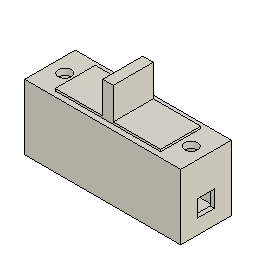
Fuse holder RT14 v0 (Autodesk Fusion 360 design; units mm, degrees)
Autodesk Fusion 360 part; units mm, degrees
sketch "Sketch1" plane through (0, 0, 0) normal (0, 0, 1) x (1, 0, 0)
  line L0 (35, -10) -> (-35, -10)
  line L1 (-35, -10) -> (-35, 10)
  line L2 (-35, 10) -> (35, 10)
  line L3 (35, 10) -> (35, -10)
  line L4 (35, -10) -> (-35, 10) construction
  line L5 (-35, -10) -> (35, 10) construction
  dimension "d1" = 70
  dimension "d2" = 20
  constraint horizontal L0
  constraint perpendicular L0 L1
  constraint parallel L0 L2
  constraint parallel L1 L3
  constraint coincident L4 origin
  constraint coincident L5 origin
  measures "d1" distance of L1.end L2.end
extrude "Extrude1" add sketch "Sketch1" along normal blind 29
sketch "Sketch2" plane through (0, 0, 0) normal (0, 0, -1) x (1, 0, 0)
  line L0 (-35, -10) -> (35, -10)
  line L1 (35, -10) -> (35, 10)
  line L2 (35, 10) -> (-35, 10)
  line L3 (-35, 10) -> (-35, -10)
  circle A0 centre (0, 0) radius 2.25
  dimension "d5" = 4.5
  constraint coincident A0.centre origin
  measures "d5" diameter of A0
shell "Shell1" thickness 2 outward yes removed faces 1 at (11.6667, -3.3333, 29)
extrude "Extrude2" cut sketch "Sketch2" along normal blind 6.615 contours A0
sketch "Sketch3" plane through (-37, 0, 0) normal (-1, 0, 0) x (0, -1, 0)
  line L0 (-12, -2) -> (12, -2)
  line L1 (12, -2) -> (12, 29)
  line L2 (12, 29) -> (-12, 29)
  line L3 (-12, 29) -> (-12, -2)
  line L4 (-4, 13) -> (4, 13)
  line L5 (4, 13) -> (4, 5)
  line L6 (4, 5) -> (-4, 5)
  line L7 (-4, 5) -> (-4, 13)
  line L8 (0, 13) -> (0, 29) construction
  dimension "d9" = 8
  dimension "d10" = 16
  constraint horizontal L4
  constraint vertical L5
  constraint horizontal L6
  constraint vertical L7
  constraint midpoint L4 L8.start
  constraint perpendicular L4 L8
  constraint equal L4 L5
  constraint midpoint L2 L8.end
  measures "d9" distance of L4.start L4.end
  measures "d10" distance of L8.start L8.end
extrude "Extrude3" cut sketch "Sketch3" against normal blind 131.311 contours L4 L5 L6 L7
sketch "Sketch4" plane through (0, 0, 29) normal (0, 0, 1) x (-1, 0, 0)
  line L0 (-35, -10) -> (-35, 10)
  line L1 (-35, 10) -> (35, 10)
  line L2 (35, 10) -> (35, -10)
  line L3 (35, -10) -> (-35, -10)
  line L4 (-37, -12) -> (37, -12)
  line L5 (37, -12) -> (37, 12)
  line L6 (37, 12) -> (-37, 12)
  line L7 (-37, 12) -> (-37, -12)
  line L8 (35, -10) -> (-35, -10)
  line L9 (-35, -10) -> (-35, 10)
  line L10 (-35, 10) -> (35, 10)
  line L11 (35, 10) -> (35, -10)
  circle A0 centre (30, 0) radius 3
  circle A1 centre (-30, 0) radius 3
  line L12 (-22, 7) -> (22, 7)
  line L13 (22, 7) -> (22, -7)
  line L14 (22, -7) -> (-22, -7)
  line L15 (-22, -7) -> (-22, 7)
  line L16 (-22, 7) -> (22, -7) construction
  line L17 (22, 7) -> (-22, -7) construction
  line L18 (30, 0) -> (-30, 0) construction
  dimension "d13" = 6
  dimension "d14" = 60
  dimension "d15" = 44
  dimension "d16" = 14
  constraint horizontal L8
  constraint vertical L9
  constraint horizontal L10
  constraint vertical L11
  constraint coincident L0.end L1.start
  constraint coincident L2.end L3.start
  constraint horizontal L12
  constraint perpendicular L12 L13
  constraint parallel L12 L14
  constraint parallel L13 L15
  constraint coincident L16 origin
  constraint coincident L17 origin
  constraint equal A0 A1
  constraint coincident A0.centre L18.start
  constraint coincident A1.centre L18.end
  constraint perpendicular L15 L18
  constraint midpoint origin L18
  measures "d13" diameter of A0
  measures "d14" distance of A0.centre A1.centre
  measures "d15" distance of L13.end L14.end
  measures "d16" distance of L12.start L14.end
extrude "Extrude4" add sketch "Sketch4" against normal blind 3 contours L0 L1 L2 L3 L8 L9 L10 L11
sketch "Sketch5" plane through (0, 0, 29) normal (0, 0, 1) x (-1, 0, 0)
  circle A0 centre (-30, 0) radius 3
  circle A1 centre (30, 0) radius 3
  line L0 (22, -7) -> (-22, -7)
  line L1 (-22, -7) -> (-22, 7)
  line L2 (-22, 7) -> (22, 7)
  line L3 (22, 7) -> (22, -7)
  line L4 (-37, -12) -> (37, -12)
  line L5 (37, -12) -> (37, 12)
  line L6 (37, 12) -> (-37, 12)
  line L7 (-37, 12) -> (-37, -12)
  line L8 (-25, 9.5) -> (25, 9.5)
  line L9 (25, 9.5) -> (25, -9.5)
  line L10 (25, -9.5) -> (-25, -9.5)
  line L11 (-25, -9.5) -> (-25, 9.5)
  line L12 (-25, 9.5) -> (25, -9.5) construction
  line L13 (25, 9.5) -> (-25, -9.5) construction
  line L14 (-2.5, 9.5) -> (2.5, 9.5)
  line L15 (2.5, 9.5) -> (2.5, -9.5)
  line L16 (2.5, -9.5) -> (-2.5, -9.5)
  line L17 (-2.5, -9.5) -> (-2.5, 9.5)
  line L18 (-2.5, 9.5) -> (2.5, -9.5) construction
  line L19 (2.5, 9.5) -> (-2.5, -9.5) construction
  dimension "d19" = 19
  dimension "d20" = 50
  dimension "d21" = 5
  constraint horizontal L8
  constraint perpendicular L8 L9
  constraint parallel L8 L10
  constraint parallel L9 L11
  constraint coincident L12 origin
  constraint coincident L13 origin
  constraint horizontal L14
  constraint perpendicular L14 L15
  constraint parallel L14 L16
  constraint parallel L15 L17
  constraint coincident L18 origin
  constraint coincident L19 origin
  constraint coincident L8 L14.start
  measures "d19" distance of L8.end L9.end
  measures "d20" distance of L9.end L10.end
  measures "d21" distance of L15 L17
extrude "Extrude5" add sketch "Sketch5" along normal blind 16 contours L0 L10 L15 L16 L17 | L0 L2 L15 L17 | L2 L8 L14 L15 L17
extrude "Extrude6" add sketch "Sketch5" along normal blind 1 contours L0 L2 L3 L8 L9 L10 L15 | L0 L2 L3 L15 | L0 L1 L2 L8 L10 L11 L17 | L0 L1 L2 L17
